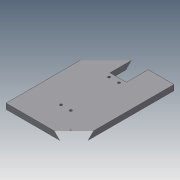
# Autodesk Inventor part: Base1
Saved by Autodesk Inventor 2014 SP1 (Build 180222100, 222)
## iProperties
Created: 2014-03-25
Part Number: Base1
Material: Generic
Document SubType Name: Modeling
Designer: tom
Density: 1 g/cm^3
Appearance: Default
Author: tom
Autodesk Inventor part; units mm, degrees
ref_plane "YZ Plane" through (0, 0, 0) normal (1, 0, 0) x (0, 1, 0)
ref_plane "XZ Plane" through (0, 0, 0) normal (0, 1, 0) x (-1, 0, 0)
ref_plane "XY Plane" through (0, 0, 0) normal (0, 0, 1) x (1, 0, 0)
sketch "Sketch1" plane through (0, 0, 0) normal (0, 1, 0) x (-1, 0, 0)
  line L0 (14, 91.5) -> (76, 91.5)
  line L1 (45, 91.5) -> (45, 1.5) construction
  circle A0 centre (49.5, 67.75) radius 1.125
  circle A1 centre (49.5, 23.75) radius 1.125
  line L2 (0, 45.75) -> (90, 45.75) construction
  circle A2 centre (40.5, 67.75) radius 1.125
  circle A3 centre (40.5, 23.75) radius 1.125
  line L3 (37.5, 20) -> (37.5, 0)
  line L4 (52.5, 20) -> (52.5, 0)
  line L5 (76, 0) -> (52.5, 0)
  line L6 (37.5, 0) -> (0, 0)
  line L7 (52.5, 20) -> (37.5, 20)
  line L8 (14, 0) -> (14, 91.5)
  line L9 (76, 0) -> (76, 91.5)
  dimension "d4" = 2.25
  dimension "d5" = 2.25
  dimension "d6" = 22
  dimension "d7" = 22
  dimension "d8" = 4.5
  dimension "d9" = 4.5
  dimension "d45" = 20
  constraints: 20 end point, 6 perpendicular, 4 centre point, 3 point on line, 2 parallel, 2 symmetric about line, 1 midpoint, 2 other
  measures "d4" diameter of A0
  measures "d5" diameter of A1
  measures "d6" distance from line of L2 A1.centre
  measures "d7" distance from line of L2 A0.centre
  measures "d8" distance from line of L1 A1.centre
  measures "d9" distance from line of A0.centre L1
  measures "d45" distance between parallel lines of L5 L7
extrude "Extrusion1" add sketch "Sketch1" along normal blind 5
sketch "Sketch4" plane through (0, 5, 0) normal (0, 1, 0) x (1, 0, 0)
  line L0 (-37.5, -20) -> (-52.5, -20) projected
  line L1 (-76, -91.5) -> (-14, -91.5) projected
  line L2 (-45, -91.5) -> (-45, -20) construction
  line L3 (-25, -83.5) -> (-14, -83.5)
  line L4 (-14, -83.5) -> (-14, -91.5)
  line L5 (-14, -91.5) -> (-25, -91.5)
  line L6 (-25, -91.5) -> (-25, -83.5)
  dimension "d28" = 11
  dimension "d29" = 8
  dimension "d30" = 0
  dimension "d31" = 20
  constraints: 10 end point, 2 midpoint, 2 parallel, 1 horizontal, 1 perpendicular
  measures "d28" distance of L4.end L5.end
  measures "d29" distance of L3.end L4.end
  measures "d30" distance between parallel lines of L1 L5
  measures "d31" distance between parallel lines of L2 L6
extrude "Extrusion4" add sketch "Sketch4" along normal blind 11
sketch "Sketch5" plane through (-14, 5, 83.5) normal (0, 0, -1) x (-1, 0, 0)
  line L0 (11, 0) -> (11, 11) projected
  line L1 (0, 11) -> (11, 11) projected
  circle A0 centre (5.5, 8) radius 1.5
  point P0 (-14, -5)
  dimension "d34" = 3
  dimension "d35" = 3
  dimension "d36" = 5.5
  constraints: 1 centre point
  measures "d34" diameter of A0
  measures "d35" distance from line of L1 A0.centre
  measures "d36" distance from line of L0 A0.centre
extrude "Extrusion5" cut sketch "Sketch5" against normal blind 8
fillet "Fillet1" radius 3 2 edges at (-14, 16, 87.5) (-25, 16, 87.5)
pattern_linear "Rectangular Pattern4" count 2 spacing 83.5 along (0, 0, -1) count 2 spacing 51 along (-1, 0, 0) of "Extrusion4", "Fillet1", "Extrusion5"
body "Solid1"
